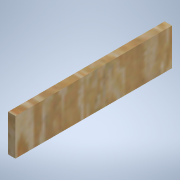
# Autodesk Inventor part: Front
Saved by Autodesk Inventor 2021.1 (Build 251245000, 245)
## iProperties
Created: 2020-08-02
Part Number: Front
Material: Default New Material(1)
Document SubType Name: Modeling
Designer: adick
Density: 1 g/cm^3
Appearance: Baltic Birch
Author: adick
Autodesk Inventor part; units mm, degrees
ref_plane "YZ Plane" through (0, 0, 0) normal (1, 0, 0) x (0, 1, 0)
ref_plane "XZ Plane" through (0, 0, 0) normal (0, 1, 0) x (-1, 0, 0)
ref_plane "XY Plane" through (0, 0, 0) normal (0, 0, 1) x (1, 0, 0)
sketch "Sketch1" plane through (0, 0, 0) normal (0, 0, 1) x (1, 0, 0)
  line L0 (135, -70.65) -> (-135, -70.65) projected
  line L1 (-135, -7) -> (-128.65, -7)
  line L2 (-128.65, -7) -> (-128.65, -70.65)
  line L3 (-128.65, -70.65) -> (-135, -70.65)
  line L4 (-135, -70.65) -> (-135, -7)
  point P0 (0, 0)
  dimension "d0" = 6.35
  constraints: 8 end point, 2 parallel, 1 horizontal, 1 perpendicular, 1 point on line, 1 other
  measures "d0" distance of L2.end L3.end
extrude "Extrusion1" add sketch "Sketch1" along normal blind 270
sketch "Sketch2" plane through (-135, -70.65, 0) normal (-1, 0, 0) x (0, 0, 1)
  line L0 (0, 63.65) -> (0, 0) projected
  line L1 (270, 63.65) -> (270, 0) projected
  line L2 (0, 63.65) -> (270, 63.65)
  line L3 (270, 63.65) -> (270, 0)
  line L4 (270, 0) -> (0, 0)
  line L5 (0, 0) -> (0, 63.65)
  point P0 (0, 70.65)
  constraints: 8 end point, 2 parallel, 1 horizontal, 1 perpendicular
extrude "Extrusion2" add sketch "Sketch2" along normal blind 6.35
sketch "Sketch3" plane through (-128.65, -7, 270) normal (0, 1, 0) x (1, 0, 0)
  line L0 (33, 330) -> (-71, 330)
  line L1 (-71, 330) -> (-71, -74)
  line L2 (-71, -74) -> (33, -74)
  line L3 (33, -74) -> (33, 330)
  point P0 (128.65, 270)
  constraints: 8 end point, 2 parallel, 1 horizontal, 1 perpendicular
extrude "Extrusion3" cut sketch "Sketch3" against normal blind 12.7
body "Solid1"
